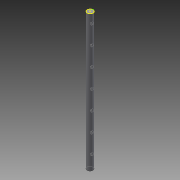
# Autodesk Inventor part: diy-rail_470mm
Saved by Autodesk Inventor 2014 (Build 180170000, 170)
## iProperties
Created: 2014-08-19
Part Number: diy-rail_470mm
Material: Generic
Document SubType Name: Modeling
Designer: Matthew
Density: 1 g/cm^3
Appearance: Default
Author: Matthew
Autodesk Inventor part; units mm, degrees
ref_plane "YZ Plane" through (0, 0, 0) normal (1, 0, 0) x (0, 1, 0)
ref_plane "XZ Plane" through (0, 0, 0) normal (0, 1, 0) x (-1, 0, 0)
sketch "Sketch1" plane through (0, 0, 0) normal (0, 0, 1) x (1, 0, 0)
  circle A0 centre (0, 0) radius 10
  dimension "d0" = 20
  constraints: 1 centre point, 1 coincident
  measures "d0" diameter of A0
extrude "Extrusion1" add sketch "Sketch1" along normal blind 470
sketch "Sketch2" plane through (0, 0, 470) normal (0, 0, 1) x (1, 0, 0)
  circle A0 centre (0, 0) radius 10 projected
  point P0 (0, 10)
  constraints: 1 vertical alignment, 1 other
ref_plane "Work Plane1" through (0, 10, 470) normal (0, 1, 0) x (-1, 0, 0)
sketch "Sketch3" plane through (0, 10, 470) normal (0, 1, 0) x (-1, 0, 0)
  line L0 (10, 0) -> (-10, 0) projected
  line L1 (0, 0) -> (0, -7.8686) construction
  point P0 (0, -470)
  point P1 (0, -40)
  point P2 (0, -105)
  point P3 (0, -170)
  point P4 (0, -235)
  point P5 (0, -300)
  point P6 (0, -365)
  point P7 (0, -430)
  dimension "d3" = 40
  dimension "d6" = 65
  dimension "d18" = 40
  constraints: 2 end point, 1 midpoint, 1 perpendicular, 1 vertical, 6 other
  measures "d3" distance from line of L0 point (0, -40)
  measures "d6" distance of point (0, -40) point (0, -105)
  measures "d18" distance of point (0, -470) point (0, -430)
hole "Hole1" at (0, 10, 430) at (0, 10, 365) at (0, 10, 300) at (0, 10, 235) at (0, 10, 170) at (0, 10, 105) at (0, 10, 40) direction (0, -1, 0) diameter 6.5278 depth 6.35
body "Solid1"
